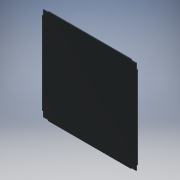
# Autodesk Inventor part: base_floor
Saved by Autodesk Inventor 2018 (Build 220112000, 112)
## iProperties
Created: 2017-10-26
Part Number: base_floor
Material: Iron, Gray
Document SubType Name: Modeling
Designer: g
Density: 7.15 g/cm^3
Appearance: Iron Gray
Author: g
Autodesk Inventor part; units mm, degrees
ref_plane "YZ Plane" through (0, 0, 0) normal (1, 0, 0) x (0, 1, 0)
ref_plane "XZ Plane" through (0, 0, 0) normal (0, 1, 0) x (-1, 0, 0)
ref_plane "XY Plane" through (0, 0, 0) normal (0, 0, 1) x (1, 0, 0)
sketch "Sketch1" plane through (0, 0, 0) normal (0, 1, 0) x (-1, 0, 0)
  line L0 (46.7, 0) -> (691.1, 0)
  line L1 (737.8, -46.7) -> (737.8, -691.1)
  line L2 (691.1, -737.8) -> (46.7, -737.8)
  line L3 (0, -691.1) -> (0, -46.7)
  line L4 (6.75, -731.05) -> (46.7, -731.05)
  line L5 (46.7, -731.05) -> (46.7, -737.8)
  line L6 (6.75, -731.05) -> (6.75, -691.1)
  line L7 (6.75, -691.1) -> (0, -691.1)
  line L8 (737.8, -691.1) -> (737.8, -368.9)
  line L9 (691.1, 0) -> (368.9, 0)
  line L10 (731.05, -731.05) -> (691.1, -731.05)
  line L11 (691.1, -731.05) -> (691.1, -737.8)
  line L12 (731.05, -731.05) -> (731.05, -691.1)
  line L13 (731.05, -691.1) -> (737.8, -691.1)
  line L14 (6.75, -6.75) -> (46.7, -6.75)
  line L15 (46.7, -6.75) -> (46.7, 0)
  line L16 (6.75, -6.75) -> (6.75, -46.7)
  line L17 (6.75, -46.7) -> (0, -46.7)
  line L18 (691.1, -6.75) -> (691.1, 0)
  line L19 (731.05, -6.75) -> (691.1, -6.75)
  line L20 (731.05, -6.75) -> (731.05, -46.7)
  line L21 (731.05, -46.7) -> (737.8, -46.7)
  point P0 (0, 0)
  point P1 (737.8, -737.8)
  point P2 (737.8, 0)
  dimension "d1" = 737.8
  dimension "d6" = 6.75
  dimension "d7" = 46.7
  dimension "d8" = 6.75
  dimension "d9" = 46.7
  dimension "d11" = 368.9
  dimension "d12" = 737.8
  dimension "d13" = 6.75
  dimension "d14" = 6.75
  dimension "d15" = 46.7
  dimension "d16" = 46.7
  constraints: 44 end point, 2 horizontal, 2 midpoint, 2 parallel, 2 perpendicular
  measures "d1" distance of point (737.8, 0) point (737.8, -737.8)
  measures "d6" distance between parallel lines of L2 L4
  measures "d7" distance between parallel lines of L3 L5
  measures "d8" distance between parallel lines of L3 L6
  measures "d9" distance between parallel lines of L2 L7
  measures "d11" distance of point (737.8, 0) L9.end
  measures "d12" distance between parallel lines of L3 L1
  measures "d13" distance between parallel lines of L1 L20
  measures "d14" distance between parallel lines of L0 L19
  measures "d15" distance between parallel lines of L0 L21
  measures "d16" distance between parallel lines of L1 L18
extrude "Extrusion1" add sketch "Sketch1" along normal blind 5
body "Solid1"
